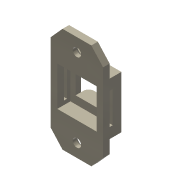
# Autodesk Inventor part: latchbase
Saved by Autodesk Inventor 2022 Beta2 (Build 260130000, 130) ContinuousBuild 0
## iProperties
Shininess: 64.0
Length Units: 11272
Angle Units: 11279
Time Units: 11290
Mass Units: 11286
Length Display Precision: 3
Angle Display Precision: 2
Created: 2002-01-23
Part Number: latchbase
Vendor: ABC Corp.
Document SubType Name: Modeling
Designer: Administrator
Density: 1 g/cm^3
Material: Generic
Appearance: Light Beige
Density: 0.0
Volumn: 0.0
Area: 0.0
PropertySet Name: Model Information
Control State: 0
Master: False
Checked Out: False
Author: Administrator
Autodesk Inventor part; units mm, degrees
ref_plane "YZ Plane" through (0, 0, 0) normal (1, 0, 0) x (0, 1, 0)
ref_plane "XZ Plane" through (0, 0, 0) normal (0, 1, 0) x (-1, 0, 0)
ref_plane "XY Plane" through (0, 0, 0) normal (0, 0, 1) x (1, 0, 0)
sketch "Sketch1" plane through (0, 0, 0) normal (0, 0, 1) x (1, 0, 0)
  line L0 (-11.6758, 23.572) -> (2.2942, 23.572)
  line L1 (2.2942, 23.572) -> (8.0092, 17.222)
  line L2 (8.0092, 17.222) -> (8.0092, -20.878)
  line L3 (8.0092, -20.878) -> (2.2942, -27.228)
  line L4 (2.2942, -27.228) -> (-11.6758, -27.228)
  line L5 (-11.6758, -27.228) -> (-17.3908, -20.878)
  line L6 (-17.3908, -20.878) -> (-17.3908, 17.222)
  line L7 (-17.3908, 17.222) -> (-11.6758, 23.572)
  line L8 (-4.6908, 23.572) -> (-4.6908, -27.228) construction
  line L9 (-17.3908, -1.828) -> (8.0092, -1.828) construction
  dimension "d0" = 25.4
  dimension "d1" = 50.8
  dimension "d2" = 5.715
  dimension "d4" = 6.35
  constraints: 20 end point, 4 equal length, 4 midpoint, 3 parallel, 2 perpendicular, 1 horizontal, 6 other
  measures "d0" distance of L1.end L6.end
  measures "d1" distance of L4.end L0.start
  measures "d2" horizontal distance of L4.end L5.end
  measures "d4" vertical distance of L4.end L5.end
extrude "Extrusion1" add sketch "Sketch1" along normal blind 3.175
sketch "Sketch2" plane through (0, 0, 3.175) normal (0, 0, 1) x (1, 0, 0)
  line L0 (-17.3908, -20.878) -> (-17.3908, 17.222) projected
  line L1 (8.0092, 17.222) -> (8.0092, -20.878) projected
  line L2 (-17.3908, 10.872) -> (8.0092, 10.872)
  line L3 (-17.3908, -14.528) -> (8.0092, -14.528)
  point P0 (2.2942, -27.228)
  dimension "d11" = 25.4
  dimension "d12" = 12.7
  constraints: 4 end point, 4 point on line, 1 parallel, 1 perpendicular
  measures "d11" distance of L2.end L3.end
  measures "d12" vertical distance of point (2.294, -27.228) L3.end
extrude "Extrusion2" add sketch "Sketch2" against normal blind 8.89
sketch "Sketch3" plane through (0, 0, -5.715) normal (0, 0, -1) x (-1, 0, 0)
  line L0 (17.3908, -14.528) -> (-8.0092, -14.528) projected
  line L1 (-8.0092, 10.872) -> (17.3908, 10.872) projected
  line L2 (-8.0092, -14.528) -> (-8.0092, 10.872) projected
  line L3 (-2.2942, 3.887) -> (11.6758, 3.887)
  line L4 (11.6758, 3.887) -> (11.6758, -7.543)
  line L5 (11.6758, -7.543) -> (-2.2942, -7.543)
  line L6 (-2.2942, -7.543) -> (-2.2942, 3.887)
  circle A0 centre (4.6908, -1.828) radius 5.715 construction
  circle A1 centre (4.6908, -1.828) radius 12.7 construction
  dimension "d15" = 11.43
  dimension "d16" = 5.715
  dimension "d17" = 5.715
  constraints: 8 end point, 5 tangent, 2 centre point, 2 parallel, 1 concentric, 1 horizontal, 1 perpendicular
  measures "d15" distance of L3.end L4.end
  measures "d16" horizontal distance of L0.end L5.end
  measures "d17" horizontal distance of L0.start L4.end
extrude "Extrusion3" cut sketch "Sketch3" against normal through all
sketch "Sketch4" plane through (0, 0, -5.715) normal (0, 0, -1) x (-1, 0, 0)
  line L0 (11.6758, 3.887) -> (11.6758, -7.543) projected
  line L1 (-2.2942, 3.887) -> (11.6758, 3.887)
  line L2 (11.6758, 3.887) -> (11.6758, 5.157)
  line L3 (11.6758, 5.157) -> (-2.2942, 5.157)
  line L4 (-2.2942, 5.157) -> (-2.2942, 3.887)
  line L5 (-2.2942, -7.543) -> (11.6758, -7.543)
  line L6 (11.6758, -7.543) -> (11.6758, -8.813)
  line L7 (11.6758, -8.813) -> (-2.2942, -8.813)
  line L8 (-2.2942, -8.813) -> (-2.2942, -7.543)
  dimension "d20" = 1.27
  dimension "d21" = 1.27
  constraints: 16 end point, 4 parallel, 2 collinear, 2 horizontal, 2 perpendicular
  measures "d20" distance of L7.end L5.start
  measures "d21" distance of L3.end L1.start
extrude "Extrusion4" add sketch "Sketch4" along normal blind 3.81
sketch "Sketch5" plane through (0, 0, 3.175) normal (0, 0, 1) x (1, 0, 0)
  line L0 (2.2942, 3.887) -> (2.2942, -7.543) projected
  line L1 (2.2942, -7.543) -> (-11.6758, -7.543) projected
  line L2 (-11.6758, -7.543) -> (-11.6758, 3.887) projected
  line L3 (-11.6758, 3.887) -> (2.2942, 3.887) projected
  line L4 (-14.2158, 7.697) -> (4.8342, 7.697)
  line L5 (4.8342, 7.697) -> (4.8342, -11.353)
  line L6 (4.8342, -11.353) -> (-14.2158, -11.353)
  line L7 (-14.2158, -11.353) -> (-14.2158, 7.697)
  point P0 (-17.3908, -20.878)
  point P1 (-11.6758, 23.572)
  dimension "d24" = 19.05
  dimension "d25" = 19.05
  dimension "d26" = 3.175
  dimension "d27" = 15.875
  constraints: 8 end point, 2 parallel, 1 horizontal, 1 perpendicular
  measures "d24" distance of L4.end L5.end
  measures "d25" distance of L5.end L6.end
  measures "d26" horizontal distance of point (-17.391, -20.878) L6.end
  measures "d27" vertical distance of point (-11.676, 23.572) L4.start
extrude "Extrusion5" cut sketch "Sketch5" against normal blind 6.35
sketch "Sketch6" plane through (-17.3908, -20.878, 3.175) normal (-1, 0, 0) x (0, 0, 1)
  line L0 (-4.699, 26.67) -> (-3.175, 26.67)
  line L1 (-3.175, 26.67) -> (-3.175, 11.43)
  line L2 (-3.175, 11.43) -> (-4.699, 11.43)
  line L3 (-4.699, 11.43) -> (-4.699, 26.67)
  line L4 (-3.175, 44.45) -> (0, 44.45) projected
  point P0 (0, 0)
  dimension "d30" = 15.24
  dimension "d31" = 1.524
  dimension "d32" = 3.175
  dimension "d33" = 17.78
  constraints: 8 end point, 2 parallel, 1 horizontal, 1 perpendicular
  measures "d30" distance of L0.end L1.end
  measures "d31" distance of L1.end L2.end
  measures "d32" horizontal distance of point (0, 0) L1.end
  measures "d33" distance from line of L0.end L4
extrude "Extrusion6" cut sketch "Sketch6" against normal through all
fillet "Fillet1" radius 2.54 4 edges at (2.2942, -8.178, -9.525) (2.2942, 4.522, -9.525) (-11.6758, 4.522, -9.525) (-11.6758, -8.178, -9.525)
sketch "Sketch7" plane through (-11.6758, -8.813, -5.715) normal (0, -1, 0) x (1, 0, 0)
  line L0 (-5.715, 5.715) -> (-5.715, 0) projected
  line L1 (0, 8.89) -> (-5.715, 8.89) projected
  point P0 (7.62, -1.905)
  dimension "d37" = 13.335
  dimension "d38" = 10.795
  measures "d37" distance from line of point (7.62, -1.905) L0
  measures "d38" distance from line of L1 point (7.62, -1.905)
hole "Hole1" at (-4.0558, -8.813, -7.62) direction (0, 1, 0) diameter 2.54 end through all
sketch "Sketch8" plane through (0, 0, 0) normal (0, 0, -1) x (-1, 0, 0)
  line L0 (-8.0092, 17.222) -> (-8.0092, 10.872) projected
  line L1 (11.6758, 23.572) -> (-2.2942, 23.572) projected
  point P0 (4.6908, 17.222)
  point P1 (4.6908, -20.878)
  dimension "d46" = 12.7
  dimension "d47" = 6.35
  dimension "d48" = 38.1
  constraints: 1 vertical alignment
  measures "d46" distance from line of point (4.691, 17.222) L0
  measures "d47" distance from line of L1 point (4.691, 17.222)
  measures "d48" distance of point (4.691, -20.878) point (4.691, 17.222)
hole "Hole2" at (-4.6908, 17.222, 0) at (-4.6908, -20.878, 0) direction (0, 0, 1) diameter 4.064 end through all countersink diameter 6.35 countersink angle 82
body "Solid1"
